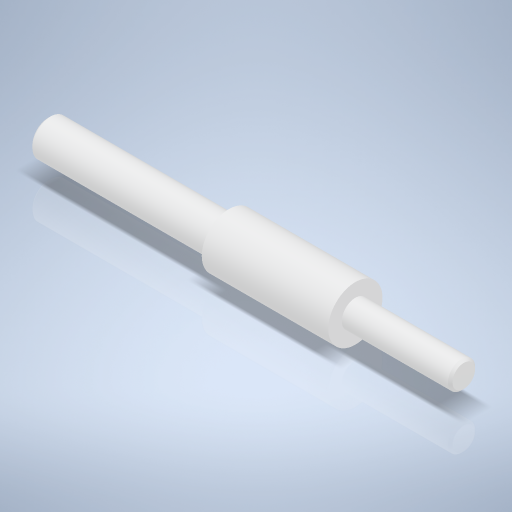
# Autodesk Inventor part: 201 Welle
Saved by Autodesk Inventor 2024 (Build 280153000, 153)
## iProperties
Created: 2024-07-12
Part Number: 201 Welle
Material: Aluminium 6061
Document SubType Name: Modeling
Designer: ffogue
Density: 2.7 g/cm^3
Appearance: Aluminium - flach
Author: ffogue
Autodesk Inventor part; units mm, degrees
ref_plane "YZ Plane" through (0, 0, 0) normal (1, 0, 0) x (0, 1, 0)
ref_plane "XZ Plane" through (0, 0, 0) normal (0, 1, 0) x (-1, 0, 0)
ref_plane "XY Plane" through (0, 0, 0) normal (0, 0, 1) x (1, 0, 0)
sketch "Skizze1" plane through (0, 0, 0) normal (0, 1, 0) x (-1, 0, 0)
  line L0 (0, 0) -> (0, 4)
  line L1 (-40, 4) -> (-40, 6)
  line L2 (-40, 6) -> (-68, 6)
  line L3 (-68, 6) -> (-68, 3)
  line L4 (-68, 3) -> (-92, 3)
  line L5 (-92, 3) -> (-92, 0)
  line L6 (-92, 0) -> (0, 0)
  line L7 (0, 4) -> (-40, 4)
  dimension "d0" = 28
  dimension "d2" = 6
  dimension "d3" = 8
  dimension "d4" = 24
  dimension "d5" = 40
  dimension "d6" = 12
  constraints: 16 end point, 5 perpendicular, 1 horizontal alignment, 1 vertical
  measures "d0" distance between parallel lines of L3 L1
  measures "d2" diameter of L4 L6
  measures "d3" diameter of L0.end L6
  measures "d4" distance between parallel lines of L5 L3
  measures "d5" distance between parallel lines of L1 L0
  measures "d6" diameter of L2 L6
revolve "Umdrehung1" add sketch "Skizze1" angle 360 about axis through (92, 0, 0) along (-1, 0, 0)
chamfer "Fasen1" distance 0.5 angle 45 2 edges at (92, 0, -3) (0, 0, -4)
